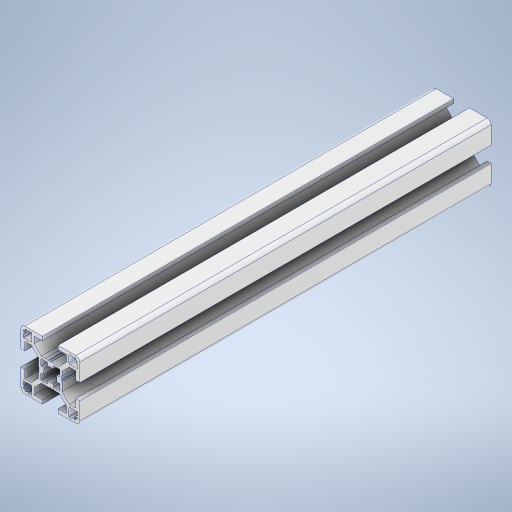
# Autodesk Inventor part: NFSL6-3030-500
Saved by Autodesk Inventor 2024 (Build 280153000, 153)
## iProperties
Category: PARTsolutions
Company: MISUMI
Created: 2024-12-13
Part Number: NFSL6-3030-500
Material: アルミニウム 6061
Catalog Web Link: www.cadenas.de
Description: NEFS6-3030, NEFSB6-3030, NEFSY6-3030, EFS6-3030, EFSB6-3030, HFS6-3030, HFSB6-3030, CAF6-3030, HFSY6-3030, NFSL6-3030,  HFSL6-3030, HFSLB6-3030, GFS6-3030-HFS6 Series Aluminum Extrusions 30 Square -1 Slot-
Vendor: MISUMI
Document SubType Name: Modeling
Designer: psAdmin
Manufacturer: MISUMI
Mass: 380.726 g
Surface Area: 1812.62 cm^2
Volume: 141.01 cm^3
Density: 2.7 g/cm^3
Appearance: アルミニウム - フラット
PSOL_IDENT_0: {$CADENAS_DATA/23d-libs/misumi/metric/38_al_extrusions_blackets/6/hfs6_3030.prj},734 {VTYP=3D},{NB=N
PSOL_IDENT_1: FSL6-3030-500},{LINA=NFSL6-3030-500},{NN=NEFS6-3030, NEFSB6-3030, NEFSY6-3030, EFS6-3030, EFSB6-3030
PSOL_IDENT_2: , HFS6-3030, HFSB6-3030, CAF6-3030, HFSY6-3030, NFSL6-3030,  HFSL6-3030, HFSLB6-3030, GFS6-3030},{DA
PSOL_IDENT_3: TE=31.05.2024 06:39:58},{GEOMDATE=16.05.2024 02:34:06},{VERSION=},{LINEID=80},{WBVAR=L,ALT1,ALT2,ALT
PSOL_IDENT_4: 3,ALT4,ALT5,CP5,DL5,DR5,ALT6,ALT9,ALT10,ALT11,DD6SE,DD6,HP6,NHL6,DL6,NHR6,DR6,ALT7,ALT8,NH9,AH,BH,CH
PSOL_IDENT_5: ,DH,EH,NH10,AV,BV,CV,DV,EV,NH11,AP,BP,CP,DP,EP,ALT12,ALT13,Z,NH12,XA,XB,XC,XD,XE,NH13,YA,YB,YC,YD,YE
PSOL_IDENT_6: ,ALT14,HP14,DL14,DR14,ALT15,HP15,DL15,DR15,ALT16,HP16,DL16,DR16,ALT17,HQ17,JLP,ALT19,ALT20},{WBNUMER
PSOL_IDENT_7: IC=L,DD6,NH9,AH,BH,CH,DH,EH,NH10,AV,BV,CV,DV,EV,NH11,AP,BP,CP,DP,EP,NH12,XA,XB,XC,XD,XE,NH13,YA,YB,Y
PSOL_IDENT_8: C,YD,YE,HQ17,JLP}  {NB=NFSL6-3030-500},{LINA=NFSL6-3030-500},{KT=DUMMY},{PN=NFSL6-3030-500},{TPS=NFS
PSOL_IDENT_9: L6-3030},{MAT=6063-T5 Aluminum Alloy},{ST=Clear Anodize},{FRMW=30},{FRMH=30},{FRD=6.8},{L=500.0},{MA
PSOL_IDENT_10: SS=0.76},{SA=280},{LX=2.68x10^4},{LY=2.68x10^4},{ALT1=},{ALT1ALG= '','w/o End Tapping', 'LTP','with
PSOL_IDENT_11: LTP (Tapping on the Left End)','RTP','with RTP (Tapping on the Right End)','LTPRTP','with LTP and RT
PSOL_IDENT_12: P (Tapping on Both Ends)','TPW','with TPW (Tapping on Both Ends)' },{M1=0},{IDM1=6.647},{DALT1=4.2},
PSOL_IDENT_13: {DPL1=0},{DPR1=0},{ALT1PN=},{ALT2=},{ALT2ALG= '','w/o End Tapping (Heli-Coil Insert)','LHP','with LH
PSOL_IDENT_14: P (Tapping on the Left (Heli-Coil Insert))','RHP','with RHP (Tapping on the Right (Heli-Coil Insert)
PSOL_IDENT_15: )','HPW','with HPW (Tapping on Both Ends (Heli-Coil Insert))' },{M2=0},{DP2=0},{ALT2PN=},{ALT3=},{AL
PSOL_IDENT_16: T3ALG= '','N/A' },{M3=0},{IDM3=4.134},{DP3=0},{ALT3PN=},{ALT4=},{ALT4ALG= '', 'w/o SC (High Precisio
PSOL_IDENT_17: n Cut)', 'SC', 'with SC (High Precision Cut)' },{ALT4PN=},{ALT5=},{ALT5ALG= '','w/o 45 Degree Cut','
PSOL_IDENT_18: 1','with 45 Degree Cut' },{CP5=},{CP5ALG= '','N/A' },{DL5=},{DL5ALG= '','N/A' },{DR5=},{DR5ALG= '','
PSOL_IDENT_19: N/A' },{FRMLALT5=0},{FRMRALT5=0},{ALT5PN=},{ALT6=},{ALT6ALG= '','w/o Fastening Location Wrench Acces
PSOL_IDENT_20: s Hole Alterations','1','with Fastening Location Wrench Access Hole Alterations' },{ALT9=},{ALT9ALG=
PSOL_IDENT_21: '','w/o Location Specified Wrench Access Hole Alteratons (Horizontal)','1','with Location Specified
PSOL_IDENT_22: Wrench Access Hole Alteratons (Horizontal)' },{ALT10=},{ALT10ALG= '','w/o Location Specified Wrench
PSOL_IDENT_23: Access Hole Alteratons (Vertical)','1','with Location Specified Wrench Access Hole Alteratons (Vert
PSOL_IDENT_24: ical)' },{ALT11=},{ALT11ALG= '','w/o Location Specified Wrench Access Hole Alteratons (Crisscross)','
PSOL_IDENT_25: 1','with Location Specified Wrench Access Hole Alteratons (Crisscross)' },{DD6SE=},{DD6SEALG= '','N/
PSOL_IDENT_26: A' },{DD6=0},{DD6ALG=0},{HP6=},{HP6ALG= '','N/A' },{NHL6=},{NHL6ALG= '','N/A' },{DL6=},{DL6ALG= '','
PSOL_IDENT_27: N/A' },{NHR6=},{NHR6ALG= '','N/A' },{DR6=},{DR6ALG= '','N/A' },{DD6PN=},{HL6=0},{HL6D=0},{HR6=0},{HR
PSOL_IDENT_28: 6D=0},{J6=0},{J6D=0},{K6=0},{K6D=0},{ALT7=},{ALT7ALG= '','N/A' },{ALT8=},{ALT8ALG= '','N/A' },{ALT67
PSOL_IDENT_29: 8PN=},{NH9=0},{NH9MAX=5},{NH9ALG=[0]},{AH=0.0},{AHMIN=7},{AHMAX=495},{AHALG=[0]},{BH=0.0},{BHMIN=2},
PSOL_IDENT_30: {BHMAX=497},{BHALG=[0]},{CH=0.0},{CHMIN=2},{CHMAX=499},{CHALG=[0]},{DH=0.0},{DHMIN=2},{DHMAX=501},{D
PSOL_IDENT_31: HALG=[0]},{EH=0.0},{EHMIN=2},{EHMAX=493},{EHALG=[0]},{NH10=0},{NH10MAX=5},{NH10ALG=[0]},{AV=0.0},{AV
PSOL_IDENT_32: MIN=7},{AVMAX=495},{AVALG=[0]},{BV=0.0},{BVMIN=2},{BVMAX=497},{BVALG=[0]},{CV=0.0},{CVMIN=2},{CVMAX=
PSOL_IDENT_33: 499},{CVALG=[0]},{DV=0.0},{DVMIN=2},{DVMAX=501},{DVALG=[0]},{EV=0.0},{EVMIN=2},{EVMAX=493},{EVALG=[0
PSOL_IDENT_34: ]},{NH11=0},{NH11MAX=5},{NH11ALG=[0]},{AP=0.0},{APMIN=7},{APMAX=495},{APALG=[0]},{BP=0.0},{BPMIN=2},
PSOL_IDENT_35: {BPMAX=497},{BPALG=[0]},{CP=0.0},{CPMIN=2},{CPMAX=499},{CPALG=[0]},{DP=0.0},{DPMIN=2},{DPMAX=501},{D
PSOL_IDENT_36: PALG=[0]},{EP=0.0},{EPMIN=2},{EPMAX=493},{EPALG=[0]},{ALT9PN=},{ALT10PN=},{ALT11PN=},{ALT91011PN=},{
PSOL_IDENT_37: ALT12=},{ALT12ALG= '','w/o Counterbore Hole in Specified Position (Vertical)','1','with Counterbore
PSOL_IDENT_38: Hole in Specified Position (Vertical)' },{ALT13=},{ALT13ALG= '','w/o Counterbore Hole in Specified P
PSOL_IDENT_39: osition (Horizontal)','1','with Counterbore Hole in Specified Position (Horizontal)' },{Z=},{ZALG= ''
PSOL_IDENT_40: ,'N/A' },{DD12=0.0},{DD112=0.0},{NH12=0},{NH12MAX=5},{NH12ALG=[0]},{XA=0.0},{XAMIN=7},{XAMAX=495},{X
PSOL_IDENT_41: AALG=[0]},{XB=0.0},{XBMIN=2},{XBMAX=497},{XBALG=[0]},{XC=0.0},{XCMIN=2},{XCMAX=499},{XCALG=[0]},{XD=
PSOL_IDENT_42: 0.0},{XDMIN=2},{XDMAX=501},{XDALG=[0]},{XE=0.0},{XEMIN=2},{XEMAX=493},{XEALG=[0]},{NH13=0},{NH13MAX=
PSOL_IDENT_43: 5},{NH13ALG=[0]},{YA=0.0},{YAMIN=7},{YAMAX=495},{YAALG=[0]},{YB=0.0},{YBMIN=2},{YBMAX=497},{YBALG=[0
PSOL_IDENT_44: ]},{YC=0.0},{YCMIN=2},{YCMAX=499},{YCALG=[0]},{YD=0.0},{YDMIN=2},{YDMAX=501},{YDALG=[0]},{YE=0.0},{Y
PSOL_IDENT_45: EMIN=2},{YEMAX=493},{YEALG=[0]},{ALT12PN=},{ALT13PN=},{ALT1213PN=},{CIFALT512=0},{CIFALT513=0},{CUTV
PSOL_IDENT_46: OLUME=1.750},{ALT14=},{ALT14ALG= '','w/o D Type Hole Alteration','1','with D Type Hole Alteration' }
PSOL_IDENT_47: ,{HP14=},{HP14ALG= '','N/A' },{DL14=},{DL14ALG= '','N/A' },{DR14=},{DR14ALG= '','N/A' },{H14=0},{D14=
PSOL_IDENT_48: 0.0},{ALT14PN=},{ALT15=},{ALT15ALG= '','w/o S Type Hole Alteration','1','with S Type Hole Alteration'
PSOL_IDENT_49: },{HP15=},{HP15ALG= '','N/A' },{DL15=},{DL15ALG= '','N/A' },{DR15=},{DR15ALG= '','N/A' },{H15=0},{D
PSOL_IDENT_50: 115=0.0},{D215=0.0},{ALT15PN=},{ALT16=},{ALT16ALG= '','w/o M Type Hole Alteration','1','with M Type
PSOL_IDENT_51: Hole Alteration' },{HP16=},{HP16ALG= '','N/A' },{DL16=},{DL16ALG= '','N/A' },{DR16=},{DR16ALG= '','N
PSOL_IDENT_52: /A' },{H116=0},{D16=0.0},{ALT16PN=},{ALT17=},{ALT17ALG= '','w/o L Type Hole Alteration (Top)','1','w
PSOL_IDENT_53: ith L Type Hole Alteration (Top)' },{HQ17=0},{HQ17ALG=0},{JLP=0},{JLPMIN=4.9},{JLPMAX=0},{JLPALG=[0]
PSOL_IDENT_54: },{L17=0},{D17=0.0},{ALT17PN=},{ALT19=},{ALT19ALG= '','N/A' },{M19=0},{DP19=0},{ALT19PN=},{ALT20=},{
PSOL_IDENT_55: ALT20PN=},{ERRORALT01=OK},{ERRORALT02=OK},{ERRORALT03=OK},{ERRORALT06091=OK},{ERRORALT05=OK},{ERRORA
PSOL_IDENT_56: LT06092=OK},{ERRORALT06093=OK},{ERRORALT06094=OK},{ERRORALT06101=OK},{ERRORALT06102=OK},{ERRORALT061
PSOL_IDENT_57: 03=OK},{ERRORALT06104=OK},{ERRORALT06111=OK},{ERRORALT06112=OK},{ERRORALT06113=OK},{ERRORALT06114=OK
PSOL_IDENT_58: },{ERRORALT06121=OK},{ERRORALT06122=OK},{ERRORALT06123=OK},{ERRORALT06124=OK},{ERRORALT06131=OK},{ER
PSOL_IDENT_59: RORALT06132=OK},{ERRORALT06133=OK},{ERRORALT06134=OK},{ERRORALT0614=OK},{ERRORALT0615=OK},{ERRORALT0
PSOL_IDENT_60: 616=OK},{ERRORALT06171=OK},{ERRORALT06172=OK},{ERRORALT06173=OK},{ERRORALT0619=OK},{ERRORALT0911=OK}
PSOL_IDENT_61: ,{ERRORALT0913=OK},{ERRORALT0914=OK},{ERRORALT0915=OK},{ERRORALT0916=OK},{ERRORALT0917=OK},{ERRORALT
PSOL_IDENT_62: 0919=OK},{ERRORALT1011=OK},{ERRORALT1012=OK},{ERRORALT1014=OK},{ERRORALT1015=OK},{ERRORALT1016=OK},{
PSOL_IDENT_63: ERRORALT1017=OK},{ERRORALT1019=OK},{ERRORALT1112=OK},{ERRORALT1113=OK},{ERRORALT1114=OK},{ERRORALT11
PSOL_IDENT_64: 15=OK},{ERRORALT1116=OK},{ERRORALT1117=OK},{ERRORALT1119=OK},{ERRORALT1214=OK},{ERRORALT1215=OK},{ER
PSOL_IDENT_65: RORALT1216=OK},{ERRORALT1217=OK},{ERRORALT1219=OK},{ERRORALT1314=OK},{ERRORALT1315=OK},{ERRORALT1316=
PSOL_IDENT_66: OK},{ERRORALT1317=OK},{ERRORALT1319=OK},{ERRORALT1415=OK},{ERRORALT1416=OK},{ERRORALT1417=OK},{ERROR
PSOL_IDENT_67: ALT1419=OK},{ERRORALT1516=OK},{ERRORALT1517=OK},{ERRORALT1519=OK},{ERRORALT1617=OK},{ERRORALT1619=OK
PSOL_IDENT_68: },{ERRORALT1719=OK},{ERRORPN=},{COLOR=},{ERRORALT01NEFSY=OK},{ERRORALT05NEFSY=OK}
NB: NFSL6-3030-500
NN: NEFS6-3030, NEFSB6-3030, NEFSY6-3030, EFS6-3030, EFSB6-3030, HFS6-3030, HFSB6-3030, CAF6-3030, HFSY6-3030, NFSL6-3030,  HFSL6-3030, HFSLB6-3030, GFS6-3030
NT: HFS6 Series Aluminum Extrusions 30 Square -1 Slot-
NBSYN: $PN.
LINA: NFSL6-3030-500
CATALOG: Misumi
PN: NFSL6-3030-500
TPS: NFSL6-3030
MAT: 6063-T5 Aluminum Alloy
ST: Clear Anodize
L: 500
MASS: 0.76
SA: 280
LX: 2.68x10^4
LY: 2.68x10^4
ALT1: w/o End Tapping
M1: 0
DPL1: 0
DPR1: 0
ALT2: w/o End Tapping (Heli-Coil Insert)
M2: 0
DP2: 0
ALT3: N/A
M3: 0
DP3: 0
ALT4: w/o SC (High Precision Cut)
ALT5: w/o 45 Degree Cut
CP5: N/A
DL5: N/A
DR5: N/A
ALT6: w/o Fastening Location Wrench Access Hole Alterations
ALT9: w/o Location Specified Wrench Access Hole Alteratons (Horizontal)
ALT10: w/o Location Specified Wrench Access Hole Alteratons (Vertical)
ALT11: w/o Location Specified Wrench Access Hole Alteratons (Crisscross)
DD6SE: N/A
DD6: 0
HP6: N/A
NHL6: N/A
DL6: N/A
NHR6: N/A
DR6: N/A
HL6D: 0
HR6D: 0
J6D: 0
K6D: 0
ALT7: N/A
ALT8: N/A
NH9: 0
AH: 0
BH: 0
CH: 0
DH: 0
EH: 0
NH10: 0
AV: 0
BV: 0
CV: 0
DV: 0
EV: 0
NH11: 0
AP: 0
BP: 0
CP: 0
DP: 0
EP: 0
ALT12: w/o Counterbore Hole in Specified Position (Vertical)
ALT13: w/o Counterbore Hole in Specified Position (Horizontal)
Z: N/A
DD12: 0
DD112: 0
NH12: 0
XA: 0
XB: 0
XC: 0
XD: 0
XE: 0
NH13: 0
YA: 0
YB: 0
YC: 0
YD: 0
YE: 0
ALT14: w/o D Type Hole Alteration
HP14: N/A
DL14: N/A
DR14: N/A
H14: 0
D14: 0
ALT15: w/o S Type Hole Alteration
HP15: N/A
DL15: N/A
DR15: N/A
H15: 0
D115: 0
D215: 0
ALT16: w/o M Type Hole Alteration
HP16: N/A
DL16: N/A
DR16: N/A
H116: 0
D16: 0
ALT17: w/o L Type Hole Alteration (Top)
HQ17: 0
JLP: 0
D17: 0
ALT19: N/A
M19: 0
DP19: 0
ALT20: w/o CW (End Face C Chamfering)
SUPPLIER: MISUMI
ARTICLENO: NFSL6-3030-500
BOMINFO: NFSL6-3030-500
CREATOR: CADENAS GmbH
Title: NFSL6-3030-500
Author: Cadenas PARTsolutions
Comments: HFS6 Series Aluminum Extrusions 30 Square -1 Slot-
Autodesk Inventor part; units mm, degrees
sketch "Sketch_118" plane through (0, 0, 0) normal (0, 0, 1) x (1, 0, 0)
  line L0 (-15, -4) -> (-15, -13)
  arc A0 (-15, -13) -> (-13, -15) centre (-13, -13) ccw
  line L1 (-13, -15) -> (-4, -15)
  line L2 (-4, -15) -> (-4, -13)
  line L3 (-4, -13) -> (-8.25, -13)
  line L4 (-8.25, -13) -> (-8.25, -9.6642)
  line L5 (-8.25, -9.6642) -> (-4.5858, -6)
  line L6 (-4.5858, -6) -> (-0.5196, -6)
  line L7 (-0.5196, -6) -> (0, -5.7)
  line L8 (0, -5.7) -> (0.4036, -5.933)
  arc A1 (0.4036, -5.933) -> (0.9036, -5.933) centre (0.6536, -5.5) ccw
  line L9 (0.9036, -5.933) -> (1.2189, -5.751)
  line L10 (1.2189, -5.751) -> (2.5, -6)
  line L11 (2.5, -6) -> (4.5858, -6)
  line L12 (4.5858, -6) -> (8.25, -9.6642)
  line L13 (8.25, -9.6642) -> (8.25, -13)
  line L14 (8.25, -13) -> (4, -13)
  line L15 (4, -13) -> (4, -15)
  line L16 (4, -15) -> (13, -15)
  arc A2 (13, -15) -> (15, -13) centre (13, -13) ccw
  line L17 (15, -13) -> (15, -4)
  line L18 (15, -4) -> (13, -4)
  line L19 (13, -4) -> (13, -8.25)
  line L20 (13, -8.25) -> (9.6642, -8.25)
  line L21 (9.6642, -8.25) -> (6, -4.5858)
  line L22 (6, -4.5858) -> (6, -0.5196)
  line L23 (6, -0.5196) -> (5.7, 0)
  line L24 (5.7, 0) -> (5.933, 0.4036)
  arc A3 (5.933, 0.4036) -> (5.933, 0.9036) centre (5.5, 0.6536) ccw
  line L25 (5.933, 0.9036) -> (5.751, 1.2189)
  line L26 (5.751, 1.2189) -> (6, 2.5)
  line L27 (6, 2.5) -> (6, 4.5858)
  line L28 (6, 4.5858) -> (9.6642, 8.25)
  line L29 (9.6642, 8.25) -> (13, 8.25)
  line L30 (13, 8.25) -> (13, 4)
  line L31 (13, 4) -> (15, 4)
  line L32 (15, 4) -> (15, 13)
  arc A4 (15, 13) -> (13, 15) centre (13, 13) ccw
  line L33 (13, 15) -> (4, 15)
  line L34 (4, 15) -> (4, 13)
  line L35 (4, 13) -> (8.25, 13)
  line L36 (8.25, 13) -> (8.25, 9.6642)
  line L37 (8.25, 9.6642) -> (4.5858, 6)
  line L38 (4.5858, 6) -> (0.5196, 6)
  line L39 (0.5196, 6) -> (0, 5.7)
  line L40 (0, 5.7) -> (-0.4036, 5.933)
  arc A5 (-0.4036, 5.933) -> (-0.9036, 5.933) centre (-0.6536, 5.5) ccw
  line L41 (-0.9036, 5.933) -> (-1.2189, 5.751)
  line L42 (-1.2189, 5.751) -> (-2.5, 6)
  line L43 (-2.5, 6) -> (-4.5858, 6)
  line L44 (-4.5858, 6) -> (-8.25, 9.6642)
  line L45 (-8.25, 9.6642) -> (-8.25, 13)
  line L46 (-8.25, 13) -> (-4, 13)
  line L47 (-4, 13) -> (-4, 15)
  line L48 (-4, 15) -> (-13, 15)
  arc A6 (-13, 15) -> (-15, 13) centre (-13, 13) ccw
  line L49 (-15, 13) -> (-15, 4)
  line L50 (-15, 4) -> (-13, 4)
  line L51 (-13, 4) -> (-13, 8.25)
  line L52 (-13, 8.25) -> (-9.6642, 8.25)
  line L53 (-9.6642, 8.25) -> (-6, 4.5858)
  line L54 (-6, 4.5858) -> (-6, 0.5196)
  line L55 (-6, 0.5196) -> (-5.7, 0)
  line L56 (-5.7, 0) -> (-5.933, -0.4036)
  arc A7 (-5.933, -0.4036) -> (-5.933, -0.9036) centre (-5.5, -0.6536) ccw
  line L57 (-5.933, -0.9036) -> (-5.751, -1.2189)
  line L58 (-5.751, -1.2189) -> (-6, -2.5)
  line L59 (-6, -2.5) -> (-6, -4.5858)
  line L60 (-6, -4.5858) -> (-9.6642, -8.25)
  line L61 (-9.6642, -8.25) -> (-13, -8.25)
  line L62 (-13, -8.25) -> (-13, -4)
  line L63 (-13, -4) -> (-15, -4)
  line L64 (9.5, -10) -> (9.5, -13.6)
  arc A8 (9.5, -13.6) -> (9.7, -13.8) centre (9.7, -13.6) ccw
  line L65 (9.7, -13.8) -> (11.2, -13.8)
  arc A9 (11.2, -13.8) -> (11.4, -13.6) centre (11.2, -13.6) ccw
  line L66 (11.4, -13.6) -> (11.4, -13.42)
  arc A10 (11.6, -13.22) -> (11.4, -13.42) centre (11.6, -13.42) ccw
  line L67 (11.6, -13.22) -> (12, -13.22)
  arc A11 (12.2, -13.42) -> (12, -13.22) centre (12, -13.42) ccw
  line L68 (12.2, -13.42) -> (12.2, -13.6)
  arc A12 (12.2, -13.6) -> (12.4, -13.8) centre (12.4, -13.6) ccw
  line L69 (12.4, -13.8) -> (12.6, -13.8)
  arc A13 (12.6, -13.8) -> (12.9, -13.5) centre (12.6, -13.5) ccw
  line L70 (12.9, -13.5) -> (12.9, -13.2)
  arc A14 (13.2, -12.9) -> (12.9, -13.2) centre (13.2, -13.2) ccw
  line L71 (13.2, -12.9) -> (13.5, -12.9)
  arc A15 (13.5, -12.9) -> (13.8, -12.6) centre (13.5, -12.6) ccw
  line L72 (13.8, -12.6) -> (13.8, -12.4)
  arc A16 (13.8, -12.4) -> (13.6, -12.2) centre (13.6, -12.4) ccw
  line L73 (13.6, -12.2) -> (13.42, -12.2)
  arc A17 (13.22, -12) -> (13.42, -12.2) centre (13.42, -12) ccw
  line L74 (13.22, -12) -> (13.22, -11.6)
  arc A18 (13.42, -11.4) -> (13.22, -11.6) centre (13.42, -11.6) ccw
  line L75 (13.42, -11.4) -> (13.6, -11.4)
  arc A19 (13.6, -11.4) -> (13.8, -11.2) centre (13.6, -11.2) ccw
  line L76 (13.8, -11.2) -> (13.8, -9.7)
  arc A20 (13.8, -9.7) -> (13.6, -9.5) centre (13.6, -9.7) ccw
  line L77 (13.6, -9.5) -> (10, -9.5)
  arc A21 (10, -9.5) -> (9.5, -10) centre (10, -10) ccw
  arc A22 (9.5, 10) -> (10, 9.5) centre (10, 10) ccw
  line L78 (10, 9.5) -> (13.6, 9.5)
  arc A23 (13.6, 9.5) -> (13.8, 9.7) centre (13.6, 9.7) ccw
  line L79 (13.8, 9.7) -> (13.8, 11.2)
  arc A24 (13.8, 11.2) -> (13.6, 11.4) centre (13.6, 11.2) ccw
  line L80 (13.6, 11.4) -> (13.42, 11.4)
  arc A25 (13.22, 11.6) -> (13.42, 11.4) centre (13.42, 11.6) ccw
  line L81 (13.22, 11.6) -> (13.22, 12)
  arc A26 (13.42, 12.2) -> (13.22, 12) centre (13.42, 12) ccw
  line L82 (13.42, 12.2) -> (13.6, 12.2)
  arc A27 (13.6, 12.2) -> (13.8, 12.4) centre (13.6, 12.4) ccw
  line L83 (13.8, 12.4) -> (13.8, 12.6)
  arc A28 (13.8, 12.6) -> (13.5, 12.9) centre (13.5, 12.6) ccw
  line L84 (13.5, 12.9) -> (13.2, 12.9)
  arc A29 (12.9, 13.2) -> (13.2, 12.9) centre (13.2, 13.2) ccw
  line L85 (12.9, 13.2) -> (12.9, 13.5)
  arc A30 (12.9, 13.5) -> (12.6, 13.8) centre (12.6, 13.5) ccw
  line L86 (12.6, 13.8) -> (12.4, 13.8)
  arc A31 (12.4, 13.8) -> (12.2, 13.6) centre (12.4, 13.6) ccw
  line L87 (12.2, 13.6) -> (12.2, 13.42)
  arc A32 (12, 13.22) -> (12.2, 13.42) centre (12, 13.42) ccw
  line L88 (12, 13.22) -> (11.6, 13.22)
  arc A33 (11.4, 13.42) -> (11.6, 13.22) centre (11.6, 13.42) ccw
  line L89 (11.4, 13.42) -> (11.4, 13.6)
  arc A34 (11.4, 13.6) -> (11.2, 13.8) centre (11.2, 13.6) ccw
  line L90 (11.2, 13.8) -> (9.7, 13.8)
  arc A35 (9.7, 13.8) -> (9.5, 13.6) centre (9.7, 13.6) ccw
  line L91 (9.5, 13.6) -> (9.5, 10)
  line L92 (-13.8, 12.6) -> (-13.8, 12.4)
  arc A36 (-13.8, 12.4) -> (-13.6, 12.2) centre (-13.6, 12.4) ccw
  line L93 (-13.6, 12.2) -> (-13.42, 12.2)
  arc A37 (-13.22, 12) -> (-13.42, 12.2) centre (-13.42, 12) ccw
  line L94 (-13.22, 12) -> (-13.22, 11.6)
  arc A38 (-13.42, 11.4) -> (-13.22, 11.6) centre (-13.42, 11.6) ccw
  line L95 (-13.42, 11.4) -> (-13.6, 11.4)
  arc A39 (-13.6, 11.4) -> (-13.8, 11.2) centre (-13.6, 11.2) ccw
  line L96 (-13.8, 11.2) -> (-13.8, 9.7)
  arc A40 (-13.8, 9.7) -> (-13.6, 9.5) centre (-13.6, 9.7) ccw
  line L97 (-13.6, 9.5) -> (-10, 9.5)
  arc A41 (-10, 9.5) -> (-9.5, 10) centre (-10, 10) ccw
  line L98 (-9.5, 10) -> (-9.5, 13.6)
  arc A42 (-9.5, 13.6) -> (-9.7, 13.8) centre (-9.7, 13.6) ccw
  line L99 (-9.7, 13.8) -> (-11.2, 13.8)
  arc A43 (-11.2, 13.8) -> (-11.4, 13.6) centre (-11.2, 13.6) ccw
  line L100 (-11.4, 13.6) -> (-11.4, 13.42)
  arc A44 (-11.6, 13.22) -> (-11.4, 13.42) centre (-11.6, 13.42) ccw
  line L101 (-11.6, 13.22) -> (-12, 13.22)
  arc A45 (-12.2, 13.42) -> (-12, 13.22) centre (-12, 13.42) ccw
  line L102 (-12.2, 13.42) -> (-12.2, 13.6)
  arc A46 (-12.2, 13.6) -> (-12.4, 13.8) centre (-12.4, 13.6) ccw
  line L103 (-12.4, 13.8) -> (-12.6, 13.8)
  arc A47 (-12.6, 13.8) -> (-12.9, 13.5) centre (-12.6, 13.5) ccw
  line L104 (-12.9, 13.5) -> (-12.9, 13.2)
  arc A48 (-13.2, 12.9) -> (-12.9, 13.2) centre (-13.2, 13.2) ccw
  line L105 (-13.2, 12.9) -> (-13.5, 12.9)
  arc A49 (-13.5, 12.9) -> (-13.8, 12.6) centre (-13.5, 12.6) ccw
  line L106 (-13.8, -12.4) -> (-13.8, -12.6)
  arc A50 (-13.8, -12.6) -> (-13.5, -12.9) centre (-13.5, -12.6) ccw
  line L107 (-13.5, -12.9) -> (-13.2, -12.9)
  arc A51 (-12.9, -13.2) -> (-13.2, -12.9) centre (-13.2, -13.2) ccw
  line L108 (-12.9, -13.2) -> (-12.9, -13.5)
  arc A52 (-12.9, -13.5) -> (-12.6, -13.8) centre (-12.6, -13.5) ccw
  line L109 (-12.6, -13.8) -> (-12.4, -13.8)
  arc A53 (-12.4, -13.8) -> (-12.2, -13.6) centre (-12.4, -13.6) ccw
  line L110 (-12.2, -13.6) -> (-12.2, -13.42)
  arc A54 (-12, -13.22) -> (-12.2, -13.42) centre (-12, -13.42) ccw
  line L111 (-12, -13.22) -> (-11.6, -13.22)
  arc A55 (-11.4, -13.42) -> (-11.6, -13.22) centre (-11.6, -13.42) ccw
  line L112 (-11.4, -13.42) -> (-11.4, -13.6)
  arc A56 (-11.4, -13.6) -> (-11.2, -13.8) centre (-11.2, -13.6) ccw
  line L113 (-11.2, -13.8) -> (-9.7, -13.8)
  arc A57 (-9.7, -13.8) -> (-9.5, -13.6) centre (-9.7, -13.6) ccw
  line L114 (-9.5, -13.6) -> (-9.5, -10)
  arc A58 (-9.5, -10) -> (-10, -9.5) centre (-10, -10) ccw
  line L115 (-10, -9.5) -> (-13.6, -9.5)
  arc A59 (-13.6, -9.5) -> (-13.8, -9.7) centre (-13.6, -9.7) ccw
  line L116 (-13.8, -9.7) -> (-13.8, -11.2)
  arc A60 (-13.8, -11.2) -> (-13.6, -11.4) centre (-13.6, -11.2) ccw
  line L117 (-13.6, -11.4) -> (-13.42, -11.4)
  arc A61 (-13.22, -11.6) -> (-13.42, -11.4) centre (-13.42, -11.6) ccw
  line L118 (-13.22, -11.6) -> (-13.22, -12)
  arc A62 (-13.42, -12.2) -> (-13.22, -12) centre (-13.42, -12) ccw
  line L119 (-13.42, -12.2) -> (-13.6, -12.2)
  arc A63 (-13.6, -12.2) -> (-13.8, -12.4) centre (-13.6, -12.4) ccw
  constraints: 240 end point, 128 point on circle, 64 centre point
extrude "Extrusion1" add sketch "Sketch_118" against normal blind 210
sketch "Sketch_94" plane through (0, 0, 0) normal (0, 0, 1) x (1, 0, 0)
  line L0 (-4.8, -1.8) -> (-4.8, -4.5)
  arc A0 (-4.8, -4.5) -> (-4.5, -4.8) centre (-4.5, -4.5) ccw
  line L1 (-4.5, -4.8) -> (-1.8, -4.8)
  arc A1 (-1.8, -4.8) -> (-1.5, -4.5) centre (-1.8, -4.5) ccw
  line L2 (-1.5, -4.5) -> (-1.5, -3.5)
  arc A2 (-1.1027, -3.2162) -> (-1.5, -3.5) centre (-1.2, -3.5) ccw
  arc A3 (-1.1027, -3.2162) -> (1.1027, -3.2162) centre (0, 0) ccw
  arc A4 (1.5, -3.5) -> (1.1027, -3.2162) centre (1.2, -3.5) ccw
  line L3 (1.5, -3.5) -> (1.5, -4.5)
  arc A5 (1.5, -4.5) -> (1.8, -4.8) centre (1.8, -4.5) ccw
  line L4 (1.8, -4.8) -> (4.5, -4.8)
  arc A6 (4.5, -4.8) -> (4.8, -4.5) centre (4.5, -4.5) ccw
  line L5 (4.8, -4.5) -> (4.8, -1.8)
  arc A7 (4.8, -1.8) -> (4.5, -1.5) centre (4.5, -1.8) ccw
  line L6 (4.5, -1.5) -> (3.5, -1.5)
  arc A8 (3.2162, -1.1027) -> (3.5, -1.5) centre (3.5, -1.2) ccw
  arc A9 (3.2162, -1.1027) -> (3.2162, 1.1027) centre (0, 0) ccw
  arc A10 (3.5, 1.5) -> (3.2162, 1.1027) centre (3.5, 1.2) ccw
  line L7 (3.5, 1.5) -> (4.5, 1.5)
  arc A11 (4.5, 1.5) -> (4.8, 1.8) centre (4.5, 1.8) ccw
  line L8 (4.8, 1.8) -> (4.8, 4.5)
  arc A12 (4.8, 4.5) -> (4.5, 4.8) centre (4.5, 4.5) ccw
  line L9 (4.5, 4.8) -> (1.8, 4.8)
  arc A13 (1.8, 4.8) -> (1.5, 4.5) centre (1.8, 4.5) ccw
  line L10 (1.5, 4.5) -> (1.5, 3.5)
  arc A14 (1.1027, 3.2162) -> (1.5, 3.5) centre (1.2, 3.5) ccw
  arc A15 (1.1027, 3.2162) -> (-1.1027, 3.2162) centre (0, 0) ccw
  arc A16 (-1.5, 3.5) -> (-1.1027, 3.2162) centre (-1.2, 3.5) ccw
  line L11 (-1.5, 3.5) -> (-1.5, 4.5)
  arc A17 (-1.5, 4.5) -> (-1.8, 4.8) centre (-1.8, 4.5) ccw
  line L12 (-1.8, 4.8) -> (-4.5, 4.8)
  arc A18 (-4.5, 4.8) -> (-4.8, 4.5) centre (-4.5, 4.5) ccw
  line L13 (-4.8, 4.5) -> (-4.8, 1.8)
  arc A19 (-4.8, 1.8) -> (-4.5, 1.5) centre (-4.5, 1.8) ccw
  line L14 (-4.5, 1.5) -> (-3.5, 1.5)
  arc A20 (-3.2162, 1.1027) -> (-3.5, 1.5) centre (-3.5, 1.2) ccw
  arc A21 (-3.2162, 1.1027) -> (-3.2162, -1.1027) centre (0, 0) ccw
  arc A22 (-3.5, -1.5) -> (-3.2162, -1.1027) centre (-3.5, -1.2) ccw
  line L15 (-3.5, -1.5) -> (-4.5, -1.5)
  arc A23 (-4.5, -1.5) -> (-4.8, -1.8) centre (-4.5, -1.8) ccw
  constraints: 48 point on circle, 32 end point, 24 centre point
extrude "Extrusion2" cut sketch "Sketch_94" against normal blind 500
ref_plane "C1_XY" through (0, 0, 0) normal (0, 0, 1) x (1, 0, 0)
ref_plane "C1_YZ" through (0, 0, 0) normal (1, 0, 0) x (0, 1, 0)
ref_plane "C1_ZX" through (0, 0, 0) normal (0, 1, 0) x (0, 0, 1)
ref_plane "to_frame_cap1_XY" through (0, 0, 0) normal (0, 0, 1) x (1, 0, 0)
ref_plane "to_frame_cap1_YZ" through (0, 0, 0) normal (1, 0, 0) x (0, 1, 0)
ref_plane "to_frame_cap1_ZX" through (0, 0, 0) normal (0, 1, 0) x (0, 0, 1)
ref_plane "to_frame_cap2_XY" through (0, 0, -500) normal (0, 0, -1) x (1, 0, 0)
ref_plane "to_frame_cap2_YZ" through (0, 0, -500) normal (1, 0, 0) x (0, -1, 0)
ref_plane "to_frame_cap2_ZX" through (0, 0, -500) normal (0, -1, 0) x (0, 0, -1)
body "Solid1"
